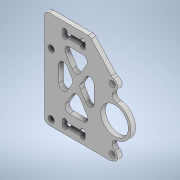
# Autodesk Inventor part: 胴体_サブフレーム_改
Saved by Autodesk Inventor 2020.4 (Build 244396000, 396)
## iProperties
Created: 2021-09-08
Part Number: 胴体_サブフレーム_改
Material: 一般
Document SubType Name: Modeling
Designer: moonk
Density: 1 g/cm^3
Appearance: 既定
Author: moonk
Autodesk Inventor part; units mm, degrees
ref_plane "YZ Plane" through (0, 0, 0) normal (1, 0, 0) x (0, 1, 0)
ref_plane "XZ Plane" through (0, 0, 0) normal (0, 1, 0) x (-1, 0, 0)
ref_plane "XY Plane" through (0, 0, 0) normal (0, 0, 1) x (1, 0, 0)
sketch "スケッチ1" plane through (0, 0, 0) normal (0, 0, 1) x (1, 0, 0)
  line L0 (-20.5, -20.49) -> (20.5, -20.49)
  line L1 (-17.5, 9.26) -> (9.5, 9.26) construction
  line L2 (9.5, 9.26) -> (9.5, -17.74) construction
  line L3 (9.5, -17.74) -> (-17.5, -17.74) construction
  line L4 (-17.5, -17.74) -> (-17.5, 9.26) construction
  circle A0 centre (-17.5, 9.26) radius 1.35
  circle A1 centre (-17.5, -17.74) radius 1.35
  circle A2 centre (9.5, -17.74) radius 1.35
  circle A3 centre (9.5, 9.26) radius 1.35
  line L5 (-14.15, 13.99) -> (1.45, 13.99)
  line L6 (1.45, 13.99) -> (1.45, -11.5897)
  line L7 (1.45, -11.5897) -> (-14.15, -11.5897)
  line L8 (-14.15, -11.5897) -> (-14.15, 13.99)
  line L9 (1.45, -9.6691) -> (-12.9787, 13.99)
  line L10 (0.2787, -11.5897) -> (-14.15, 12.0694)
  line L11 (1.4958, 12.1446) -> (-12.9787, -11.5897)
  line L12 (0.0396, 13.99) -> (-14.15, -9.2771)
  circle A4 centre (9.5, 9.26) radius 2.35 construction
  arc A5 (9.5, 6.91) -> (9.5, 11.61) centre (9.5, 9.26) ccw
  circle A6 centre (9.5, -17.74) radius 2.35 construction
  line L13 (9.5, -20.09) -> (9.5, -20.49)
  arc A7 (9.5, -20.09) -> (9.5, -15.39) centre (9.5, -17.74) ccw
  circle A8 centre (10.5, -4.24) radius 6.05
  circle A9 centre (10.5, -4.24) radius 7.25 construction
  line L14 (9.5, 6.91) -> (9.5, 2.9407)
  line L15 (9.5, -11.4207) -> (9.5, -15.39)
  arc A10 (9.5, -11.4207) -> (9.5, 2.9407) centre (10.5, -4.24) ccw
  line L16 (-12.5, 19.03) -> (-12.51, 19.03)
  line L17 (-12.51, 19.03) -> (-2.49, 19.03)
  line L18 (-2.49, 19.03) -> (-2.49, 17.01)
  line L19 (-2.49, 17.01) -> (-12.51, 17.01)
  line L20 (-12.51, 17.01) -> (-12.51, 19.03)
  line L21 (-20.5, 22.49) -> (20.5, 22.49)
  line L22 (-0.3631, 22.49) -> (9.5, 11.61)
  line L23 (-20.5, 22.49) -> (-20.5, -20.49)
  line L24 (20.5, 22.49) -> (20.5, -20.49)
  circle A11 centre (-11.46, 19.03) radius 1.05
  circle A12 centre (-11.46, 17.01) radius 1.05
  circle A13 centre (-3.54, 19.03) radius 1.05
  circle A14 centre (-3.54, 17.01) radius 1.05
  line L25 (-12.51, -15.49) -> (-2.49, -15.49)
  line L26 (-2.49, -15.49) -> (-2.49, -17.51)
  line L27 (-2.49, -17.51) -> (-12.51, -17.51)
  line L28 (-12.51, -17.51) -> (-12.51, -15.49)
  circle A15 centre (-11.46, -17.51) radius 1.05
  circle A16 centre (-3.54, -15.49) radius 1.05
  circle A17 centre (-3.54, -17.51) radius 1.05
  circle A18 centre (-11.46, -15.49) radius 1.05
  point P0 (0, 0)
  point P1 (-5.1787, 1.2001)
  point P2 (1.45, 12.0694)
  point P3 (-6.35, -0.7205)
  point P4 (-7.6408, 1.3962)
  point P5 (-6.4695, 3.3167)
  point P6 (-4.59, 17.01)
  point P7 (-10.41, 17.01)
  point P8 (-10.41, 19.03)
  point P9 (-4.59, 19.03)
  point P10 (-4.59, -17.51)
  point P11 (-10.41, -17.51)
  point P12 (-10.41, -15.49)
  point P13 (-4.59, -15.49)
  dimension "d184" = 2.1
  dimension "d186" = 2.1
  dimension "d210" = 2.1
  dimension "d211" = 2.1
  dimension "d212" = 2.1
  dimension "d213" = 2.1
  dimension "d12" = 27
  dimension "d22" = 27
  dimension "d24" = 2.7
  dimension "d26" = 2.7
  dimension "d27" = 2.7
  dimension "d28" = 2.7
  dimension "d72" = 15.6
  dimension "d73" = 25.5797
  dimension "d87" = 4.7
  dimension "d88" = 4.7
  dimension "d96" = 12.1
  dimension "d97" = 14.5
  dimension "d99" = 16.25
  dimension "d160" = 10.02
  dimension "d165" = 42.98
  dimension "d166" = 41
  dimension "d167" = 20.5
  dimension "d168" = 20.5
  dimension "d169" = 22.49
  dimension "d170" = 47.807
  dimension "d171" = 10.88
  dimension "d172" = 13.99
  dimension "d173" = 1.45
  dimension "d174" = 9.26
  dimension "d175" = 17.5
  dimension "d176" = 10.5
  dimension "d178" = 7.99
  dimension "d179" = 17.01
  dimension "d180" = 2.02
  dimension "d183" = 2.1
  dimension "d185" = 2.1
  dimension "d187" = 9.04
  dimension "d188" = 3.54
  dimension "d205" = 10.02
  dimension "d206" = 2.02
  dimension "d207" = 5
  dimension "d208" = 7.99
  constraints: 58 end point, 21 point on line, 13 centre point, 12 point on circle, 9 parallel, 7 coincident, 5 horizontal, 5 perpendicular, 3 concentric, 1 collinear, 1 vertical, 22 other
  measures "d12" distance of L2.end L3.end
  measures "d22" distance of L1.end L2.end
  measures "d24" diameter of A0
  measures "d26" diameter of A3
  measures "d27" diameter of A1
  measures "d28" diameter of A2
  measures "d72" distance of L5.start L5.end
  measures "d73" distance of L7.end L5.start
  measures "d87" diameter of A4
  measures "d88" diameter of A6
  measures "d96" diameter of A8
  measures "d97" diameter of A9
  measures "d99" distance from line of L0 A8.centre
  measures "d160" distance of L18.end L19.end
  measures "d165" distance of L21.start L0.start
  measures "d166" distance of L21.start L21.end
  measures "d167" distance from line of L24 point (0, 0)
  measures "d168" distance from line of point (0, 0) L23
  measures "d169" distance from line of L21 point (0, 0)
  measures "d170" angle of L22 L21
  measures "d171" vertical distance of L22.start L22.end
  measures "d172" distance from line of point (0, 0) L5
  measures "d173" distance from line of L6 point (0, 0)
  measures "d174" distance from line of point (0, 0) L1
  measures "d175" distance from line of point (0, 0) L4
  measures "d176" horizontal distance of point (0, 0) A8.centre
  measures "d178" distance between parallel lines of L23 L20
  measures "d179" distance from line of point (0, 0) L19
  measures "d180" distance between parallel lines of L19 L17
  measures "d183" diameter of A11
  measures "d185" diameter of A13
  measures "d187" distance from line of L23 A11.centre
  measures "d188" horizontal distance of point (0, 0) A13.centre
  measures "d205" distance of L26.end L27.end
  measures "d206" distance of L25.end L26.end
  measures "d207" distance between parallel lines of L0 L25
  measures "d208" distance between parallel lines of L23 L28
extrude "押し出し1" add sketch "スケッチ1" along normal blind 2 contours L23 L21 L22 A5 L14 A10 L15 A7 L13 L0 | L5 L9 L12 L10 L8 | L5 L6 L11 L9 L12 | L9 L11 L10 L12 | L12 L10 L11 L7 L8 | L9 L6 L7 L10 L11
fillet "フィレット4" radius 2 12 edges at (-12.9787, 13.99, 1) (0.0396, 13.99, 1) (1.45, 12.0694, 1) (-6.35, -0.7205, 1) (-5.1787, 1.2001, 1) (-7.6408, 1.3962, 1) (-6.4695, 3.3167, 1) (-14.15, 12.0694, 1) (-14.15, -9.2771, 1) (-12.9787, -11.5897, 1) (0.2787, -11.5897, 1) (1.45, -9.6691, 1)
fillet "フィレット5" radius 2 9 edges at (-20.5, 22.49, 1) (-0.3631, 22.49, 1) (9.5, 11.61, 1) (9.5, 6.91, 1) (9.5, 2.9407, 1) (9.5, -11.4207, 1) (9.5, -15.39, 1) (-20.5, -20.49, 1) (9.5, -20.49, 1)
equation "\"d22\" = d12"
equation "\"d26\" = d24"
equation "\"d27\" = d24"
equation "\"d28\" = d24"
